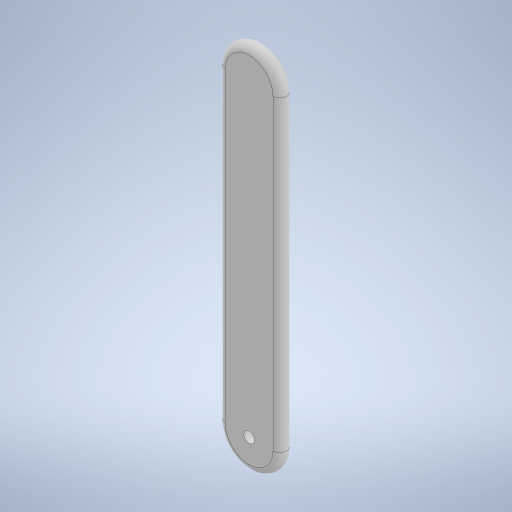
# Autodesk Inventor part: шатун22
Saved by Autodesk Inventor 2023.1 (Build 271208000, 208)
## iProperties
Created: 2024-12-17
Part Number: шатун22
Material: Типовые
Document SubType Name: Modeling
Designer: DELL
Density: 1 g/cm^3
Appearance: По умолчанию
Author: DELL
Autodesk Inventor part; units mm, degrees
ref_plane "YZ Plane" through (0, 0, 0) normal (1, 0, 0) x (0, 1, 0)
ref_plane "XZ Plane" through (0, 0, 0) normal (0, 1, 0) x (-1, 0, 0)
ref_plane "XY Plane" through (0, 0, 0) normal (0, 0, 1) x (1, 0, 0)
sketch "Эскиз1" plane through (0, 0, 0) normal (0, 0, 1) x (1, 0, 0)
  circle A0 centre (0, 0) radius 9
  circle A1 centre (0, 0) radius 1.575
  line L0 (0, -9) -> (0, 99) construction
  line L1 (-9, 0) -> (-9, 90)
  line L2 (9, 90) -> (9, 0)
  arc A2 (-9, 0) -> (9, 0) centre (0, 0) ccw
  arc A3 (9, 90) -> (-9, 90) centre (0, 90) ccw
  point P0 (0, 45)
  dimension "d0" = 18
  dimension "d1" = 3.15
  dimension "d5" = 108
  constraints: 8 end point, 6 point on circle, 4 tangent, 3 centre point, 2 coincident, 2 point on line, 1 midpoint, 1 parallel, 1 vertical, 3 other
  measures "d1" diameter of A1
  measures "d5" distance of L0.start L0.end
extrude "Выдавливание1" add sketch "Эскиз1" along normal blind 4
fillet "Сопряжение1" radius 2 8 edges at (0, 99, 0) (-9, 45, 0) (0, -9, 0) (9, 45, 0) (0, -9, 4) (9, 45, 4) (0, 99, 4) (-9, 45, 4)
sketch "Эскиз2" plane through (0, 0, 0) normal (0, 0, -1) x (-1, 0, 0)
  line L0 (-3.1902, 30.8529) -> (-3.1902, 57.702) construction
  line L1 (-3.1902, 57.702) -> (13.4433, 57.702) construction
  line L2 (13.4433, 57.702) -> (13.4433, 30.8529) construction
  line L3 (13.4433, 30.8529) -> (-3.1902, 30.8529) construction
  line L4 (-0.1402, 36.9062) -> (2.4592, 36.9062)
  line L5 (2.4592, 36.9062) -> (2.4592, 38.8605)
  spline S0 degree 2 poles (2.4592, 38.8605) (2.4592, 39.0739) (2.6726, 39.0739) knots 0 0 0 1 1 1
  spline S1 degree 2 poles (2.6726, 39.0739) (2.8908, 39.0739) (2.8908, 38.8605) knots 0 0 0 1 1 1
  line L6 (2.8908, 38.8605) -> (2.8908, 36.6928)
  spline S2 degree 2 poles (2.8908, 36.6928) (2.8908, 36.4746) (2.6726, 36.4746) knots 0 0 0 1 1 1
  line L7 (2.6726, 36.4746) -> (-2.9625, 36.4746)
  spline S3 degree 2 poles (-2.9625, 36.4746) (-3.1807, 36.4746) (-3.1807, 36.6928) knots 0 0 0 1 1 1
  line L8 (-3.1807, 36.6928) -> (-3.1807, 38.8605)
  spline S4 degree 2 poles (-3.1807, 38.8605) (-3.1807, 39.0739) (-2.9673, 39.0739) knots 0 0 0 1 1 1
  spline S5 degree 2 poles (-2.9673, 39.0739) (-2.7491, 39.0739) (-2.7491, 38.8605) knots 0 0 0 1 1 1
  line L9 (-2.7491, 38.8605) -> (-2.7491, 36.9062)
  line L10 (-2.7491, 36.9062) -> (-0.5719, 36.9062)
  line L11 (-0.5719, 36.9062) -> (-0.5719, 37.9924)
  spline S6 degree 2 poles (-0.5719, 37.9924) (-0.5719, 38.2059) (-0.3584, 38.2059) knots 0 0 0 1 1 1
  spline S7 degree 2 poles (-0.3584, 38.2059) (-0.1402, 38.2059) (-0.1402, 37.9924) knots 0 0 0 1 1 1
  line L12 (-0.1402, 37.9924) -> (-0.1402, 36.9062)
  spline S8 degree 2 poles (3.9438, 40.3736) (4.3138, 40.3736) (4.8356, 39.8613) (4.8356, 39.4961) knots 0 0 0 1 2 2 2
  line L13 (4.8356, 39.4961) -> (4.8356, 39.2684)
  spline S9 degree 2 poles (4.8356, 39.2684) (4.8356, 39.0502) (4.6174, 39.0502) knots 0 0 0 1 1 1
  spline S10 degree 2 poles (4.6174, 39.0502) (4.4466, 39.0502) (4.4134, 39.2068) knots 0 0 0 1 1 1
  spline S11 degree 2 poles (4.4134, 39.2068) (4.3992, 39.2494) (4.3992, 39.4961) knots 0 0 0 1 1 1
  spline S12 degree 2 poles (4.3992, 39.4961) (4.3992, 39.6811) (4.1336, 39.942) (3.9438, 39.942) knots 0 0 0 1 2 2 2
  line L14 (3.9438, 39.942) -> (-1.1885, 39.942)
  spline S13 degree 2 poles (-1.1885, 39.942) (-1.402, 39.942) (-1.402, 40.1602) knots 0 0 0 1 1 1
  spline S14 degree 2 poles (-1.402, 40.1602) (-1.402, 40.3736) (-1.1885, 40.3736) knots 0 0 0 1 1 1
  line L15 (-1.1885, 40.3736) -> (3.9438, 40.3736)
  spline S15 degree 2 poles (-2.7491, 40.1602) (-2.7491, 39.9372) (-2.972, 39.9372) knots 0 0 0 1 1 1
  spline S16 degree 2 poles (-2.972, 39.9372) (-3.1902, 39.9372) (-3.1902, 40.1602) knots 0 0 0 1 1 1
  spline S17 degree 2 poles (-3.1902, 40.1602) (-3.1902, 40.3831) (-2.972, 40.3831) knots 0 0 0 1 1 1
  spline S18 degree 2 poles (-2.972, 40.3831) (-2.7491, 40.3831) (-2.7491, 40.1602) knots 0 0 0 1 1 1
  line L16 (0.9413, 41.6686) -> (2.0275, 41.6686)
  spline S19 degree 2 poles (2.0275, 41.6686) (2.203, 41.6686) (2.4592, 41.92) (2.4592, 42.1002) knots 0 0 0 1 2 2 2
  line L17 (2.4592, 42.1002) -> (2.4592, 43.6228)
  spline S20 degree 2 poles (2.4592, 43.6228) (2.4592, 43.841) (2.6726, 43.841) knots 0 0 0 1 1 1
  spline S21 degree 2 poles (2.6726, 43.841) (2.8908, 43.841) (2.8908, 43.6228) knots 0 0 0 1 1 1
  line L18 (2.8908, 43.6228) -> (2.8908, 42.1002)
  spline S22 degree 2 poles (2.8908, 42.1002) (2.8908, 41.7397) (2.3833, 41.2369) (2.0228, 41.2369) knots 0 0 0 1 2 2 2
  line L19 (2.0228, 41.2369) -> (-0.5719, 41.2369)
  spline S23 degree 2 poles (-0.5719, 41.2369) (-0.9276, 41.2369) (-1.4399, 41.7445) (-1.4399, 42.1002) knots 0 0 0 1 2 2 2
  line L20 (-1.4399, 42.1002) -> (-1.4399, 42.9777)
  spline S24 degree 2 poles (-1.4399, 42.9777) (-1.4399, 43.3382) (-0.9324, 43.8458) (-0.5719, 43.8458) knots 0 0 0 1 2 2 2
  line L21 (-0.5719, 43.8458) -> (0.7231, 43.8458)
  spline S25 degree 2 poles (0.7231, 43.8458) (0.9413, 43.8458) (0.9413, 43.6228) knots 0 0 0 1 1 1
  line L22 (0.9413, 43.6228) -> (0.9413, 41.6686)
  line L23 (0.5096, 41.6686) -> (0.5096, 43.4141)
  line L24 (0.5096, 43.4141) -> (-0.5766, 43.4141)
  spline S26 degree 2 poles (-0.5766, 43.4141) (-0.7521, 43.4141) (-1.0083, 43.158) (-1.0083, 42.9777) knots 0 0 0 1 2 2 2
  line L25 (-1.0083, 42.9777) -> (-1.0083, 42.1002)
  spline S27 degree 2 poles (-1.0083, 42.1002) (-1.0083, 41.92) (-0.7521, 41.6686) (-0.5766, 41.6686) knots 0 0 0 1 2 2 2
  line L26 (-0.5766, 41.6686) -> (0.5096, 41.6686)
  spline S28 degree 2 poles (2.6726, 47.3179) (2.8908, 47.3179) (2.8908, 47.1045) knots 0 0 0 1 1 1
  spline S29 degree 2 poles (2.8908, 47.1045) (2.8908, 46.8863) (2.6726, 46.8863) knots 0 0 0 1 1 1
  line L27 (2.6726, 46.8863) -> (-0.5814, 46.8863)
  spline S30 degree 2 poles (-0.5814, 46.8863) (-0.7616, 46.8863) (-1.0178, 46.6302) (-1.0178, 46.4499) knots 0 0 0 1 2 2 2
  line L28 (-1.0178, 46.4499) -> (-1.0178, 45.1407)
  line L29 (-1.0178, 45.1407) -> (2.6726, 45.1407)
  spline S31 degree 2 poles (2.6726, 45.1407) (2.8908, 45.1407) (2.8908, 44.9273) knots 0 0 0 1 1 1
  spline S32 degree 2 poles (2.8908, 44.9273) (2.8908, 44.7091) (2.6726, 44.7091) knots 0 0 0 1 1 1
  line L30 (2.6726, 44.7091) -> (-1.2312, 44.7091)
  spline S33 degree 2 poles (-1.2312, 44.7091) (-1.4494, 44.7091) (-1.4494, 44.9273) knots 0 0 0 1 1 1
  line L31 (-1.4494, 44.9273) -> (-1.4494, 46.4499)
  spline S34 degree 2 poles (-1.4494, 46.4499) (-1.4494, 46.8057) (-0.9371, 47.3179) (-0.5814, 47.3179) knots 0 0 0 1 2 2 2
  line L32 (-0.5814, 47.3179) -> (2.6726, 47.3179)
  line L33 (-1.236, 48.6176) -> (2.6726, 48.6176)
  spline S35 degree 2 poles (2.6726, 48.6176) (2.8908, 48.6176) (2.8908, 48.4042) knots 0 0 0 1 1 1
  spline S36 degree 2 poles (2.8908, 48.4042) (2.8908, 48.1907) (2.6726, 48.1907) knots 0 0 0 1 1 1
  line L34 (2.6726, 48.1907) -> (-1.236, 48.1907)
  spline S37 degree 2 poles (-1.236, 48.1907) (-1.4494, 48.1907) (-1.4494, 48.4042) knots 0 0 0 1 1 1
  spline S38 degree 2 poles (-1.4494, 48.4042) (-1.4494, 48.6176) (-1.236, 48.6176) knots 0 0 0 1 1 1
  spline S39 degree 2 poles (-3.1807, 48.4042) (-3.1807, 48.6176) (-2.9625, 48.6176) knots 0 0 0 1 1 1
  spline S40 degree 2 poles (-2.9625, 48.6176) (-2.7491, 48.6176) (-2.7491, 48.4042) knots 0 0 0 1 1 1
  spline S41 degree 2 poles (-2.7491, 48.4042) (-2.7491, 48.186) (-2.9625, 48.186) knots 0 0 0 1 1 1
  spline S42 degree 2 poles (-2.9625, 48.186) (-3.1807, 48.186) (-3.1807, 48.4042) knots 0 0 0 1 1 1
  line L35 (0.9413, 49.9126) -> (2.0275, 49.9126)
  spline S43 degree 2 poles (2.0275, 49.9126) (2.203, 49.9126) (2.4592, 50.164) (2.4592, 50.3442) knots 0 0 0 1 2 2 2
  line L36 (2.4592, 50.3442) -> (2.4592, 51.8669)
  spline S44 degree 2 poles (2.4592, 51.8669) (2.4592, 52.0851) (2.6726, 52.0851) knots 0 0 0 1 1 1
  spline S45 degree 2 poles (2.6726, 52.0851) (2.8908, 52.0851) (2.8908, 51.8669) knots 0 0 0 1 1 1
  line L37 (2.8908, 51.8669) -> (2.8908, 50.3442)
  spline S46 degree 2 poles (2.8908, 50.3442) (2.8908, 49.9837) (2.3833, 49.4809) (2.0228, 49.4809) knots 0 0 0 1 2 2 2
  line L38 (2.0228, 49.4809) -> (-0.5719, 49.4809)
  spline S47 degree 2 poles (-0.5719, 49.4809) (-0.9276, 49.4809) (-1.4399, 49.9885) (-1.4399, 50.3442) knots 0 0 0 1 2 2 2
  line L39 (-1.4399, 50.3442) -> (-1.4399, 51.2218)
  spline S48 degree 2 poles (-1.4399, 51.2218) (-1.4399, 51.5823) (-0.9324, 52.0898) (-0.5719, 52.0898) knots 0 0 0 1 2 2 2
  line L40 (-0.5719, 52.0898) -> (0.7231, 52.0898)
  spline S49 degree 2 poles (0.7231, 52.0898) (0.9413, 52.0898) (0.9413, 51.8669) knots 0 0 0 1 1 1
  line L41 (0.9413, 51.8669) -> (0.9413, 49.9126)
  line L42 (0.5096, 49.9126) -> (0.5096, 51.6582)
  line L43 (0.5096, 51.6582) -> (-0.5766, 51.6582)
  spline S50 degree 2 poles (-0.5766, 51.6582) (-0.7521, 51.6582) (-1.0083, 51.402) (-1.0083, 51.2218) knots 0 0 0 1 2 2 2
  line L44 (-1.0083, 51.2218) -> (-1.0083, 50.3442)
  spline S51 degree 2 poles (-1.0083, 50.3442) (-1.0083, 50.164) (-0.7521, 49.9126) (-0.5766, 49.9126) knots 0 0 0 1 2 2 2
  line L45 (-0.5766, 49.9126) -> (0.5096, 49.9126)
  point P0 (0, 0)
  constraints: 2 other
emboss "Рельеф1" sketch "Эскиз2" operation cut depth 2 direction (0, 0, 1)
